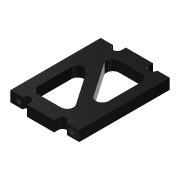
# Autodesk Inventor part: 前腕_サブフレーム_1_1
Saved by Autodesk Inventor 2017.3 (Build 213256000, 256)
## iProperties
Created: 2016-05-04
Part Number: 前腕_サブフレーム_1_1
Material: アセタール樹脂、黒
Document SubType Name: Modeling
Designer: hiroaki
Density: 1.425 g/cm^3
Appearance: 滑らか - 黒
Mass: 16.6655 g
Surface Area: 81.5563 cm^2
Volume: 11.6951 cm^3
Author: hiroaki
Autodesk Inventor part; units mm, degrees
ref_plane "YZ Plane" through (0, 0, 0) normal (1, 0, 0) x (0, 1, 0)
ref_plane "XZ Plane" through (0, 0, 0) normal (0, 1, 0) x (-1, 0, 0)
ref_plane "XY Plane" through (0, 0, 0) normal (0, 0, 1) x (1, 0, 0)
sketch "スケッチ1" plane through (0, 0, 0) normal (0, 0, 1) x (1, 0, 0)
  line L0 (-16.5, -21.65) -> (16.5, -21.65) construction
  line L1 (16.5, -21.65) -> (16.5, 21.65) construction
  line L2 (16.5, 21.65) -> (-16.5, 21.65) construction
  line L3 (-16.5, 21.65) -> (-16.5, -21.65) construction
  line L4 (-16.5, -21.65) -> (16.5, 21.65) construction
  line L5 (16.5, -21.65) -> (-16.5, 21.65) construction
  line L6 (-12.5, 21.65) -> (-12.5, -21.65) construction
  line L7 (0, 0) -> (0, 21.65) construction
  line L8 (0, 0) -> (-16.5, 0) construction
  line L9 (12.5, 21.65) -> (12.5, -21.65) construction
  line L10 (-16.5, -21.65) -> (-10.6, -21.65)
  line L11 (-6.5, 21.65) -> (-6.5, 23.65)
  line L12 (-6.5, 23.65) -> (6.5, 23.65)
  line L13 (6.5, 23.65) -> (6.5, 21.65)
  line L14 (10.6, 21.65) -> (16.5, 21.65)
  line L15 (16.5, 21.65) -> (16.5, -21.65)
  line L16 (16.5, -21.65) -> (10.6, -21.65)
  line L17 (-6.5, -21.65) -> (-6.5, -23.65)
  line L18 (-6.5, -23.65) -> (6.5, -23.65)
  line L19 (6.5, -23.65) -> (6.5, -21.65)
  arc A0 (-10.6, 21.65) -> (-6.5, 21.65) centre (-8.55, 21.65) ccw
  arc A1 (6.5, 21.65) -> (10.6, 21.65) centre (8.55, 21.65) ccw
  arc A2 (-6.5, -21.65) -> (-10.6, -21.65) centre (-8.55, -21.65) ccw
  arc A3 (10.6, -21.65) -> (6.5, -21.65) centre (8.55, -21.65) ccw
  line L20 (-16.5, -21.65) -> (-16.5, -16.65)
  line L21 (-16.5, -16.65) -> (-16.5, 21.65)
  line L22 (-10.6, 21.65) -> (-16.5, 21.65)
  line L23 (6.95, 24.476) -> (10.05, 24.476) construction
  line L24 (10.05, 24.476) -> (10.05, 13.3235) construction
  line L25 (10.05, 13.3235) -> (6.95, 13.3235) construction
  line L26 (6.95, 13.3235) -> (6.95, 24.476) construction
  line L27 (8.5, 24.476) -> (8.5, 13.3235) construction
  line L28 (-18.05, 24.476) -> (-14.95, 24.476) construction
  line L29 (-14.95, 24.476) -> (-14.95, 13.9945) construction
  line L30 (-14.95, 13.9945) -> (-18.05, 13.9945) construction
  line L31 (-18.05, 13.9945) -> (-18.05, 24.476) construction
  line L32 (-16.5, 24.476) -> (-16.5, 13.9945) construction
  dimension "d16" = 4
  dimension "d20" = 43.3
  dimension "d40" = 25
  dimension "d41" = 6
  dimension "d42" = 2.05
  dimension "d43" = 2
  dimension "d44" = 5
  dimension "d48" = 3.1
  dimension "d51" = 25
  dimension "d52" = 3.1
  dimension "d81" = 6
  constraints: 66 end point, 11 perpendicular, 8 midpoint, 8 point on circle, 6 parallel, 6 point on line, 5 collinear, 4 centre point, 4 horizontal, 4 horizontal alignment, 3 equal radius, 3 tangent, 2 symmetric about line, 2 vertical, 4 other
  measures "d16" distance between parallel lines of L3 L6
  measures "d20" distance of L2.end L0.start
  measures "d40" distance between parallel lines of L9 L6
  measures "d41" distance between parallel lines of L6 L17
  measures "d42" radius of A2
  measures "d43" distance between parallel lines of L0 L18
  measures "d44" distance from line of L10 L20.end
  measures "d48" distance of L23.start L23.end
  measures "d51" distance between parallel lines of L27 L32
  measures "d52" distance of L28.start L28.end
  measures "d81" distance between parallel lines of L11 L6
extrude "押し出し1" add sketch "スケッチ1" along normal blind 2.5
mirror "ミラー1" about plane through (0, 0, 0) normal (0, 0, -1) of "押し出し1"
sketch "スケッチ2" plane through (-16.5, -21.65, 2.5) normal (0, -1, 0) x (1, 0, 0)
  line L0 (0, -5) -> (0, 0)
  line L1 (10, -5) -> (23, -5) construction
  line L2 (16.5, -5) -> (16.5, 0) construction
  line L3 (10, 0) -> (23, 0) construction
  point P0 (16.5, -2.5)
  point P1 (4, -2.5)
  point P2 (29, -2.5)
  point P3 (0, -2.5)
  dimension "d26" = 4
  constraints: 4 end point, 3 midpoint, 2 horizontal alignment, 1 symmetric about line
  measures "d26" distance from line of point (4, -2.5) L0
hole "穴1" at (-12.5, -21.65, 0) at (12.5, -21.65, 0) direction (0, 1, 0) diameter 2.459 depth 2 thread size "M3x0.5" class "6H" standard "ISO Metric profile"
sketch "スケッチ4" plane through (10.6, 21.65, 2.5) normal (0, 1, 0) x (1, 0, 0)
  line L0 (5.9, 5) -> (5.9, 0) projected
  point P0 (-10.6, 2.5)
  point P1 (1.9, 2.5)
  point P2 (-23.1, 2.5)
  point P3 (5.9, 2.5)
  dimension "d53" = 4
  dimension "d54" = 25
  constraints: 2 horizontal alignment, 1 midpoint
  measures "d53" distance from line of point (1.9, 2.5) L0
  measures "d54" distance of point (-23.1, 2.5) point (1.9, 2.5)
hole "穴2" at (12.5, 21.65, 0) at (-12.5, 21.65, 0) direction (0, -1, 0) diameter 2.459 depth 2.5 thread size "M3x0.5" class "6H" standard "ISO Metric profile"
sketch "スケッチ6" plane through (0, 0, 2.5) normal (0, 0, 1) x (1, 0, 0)
  line L0 (10.6, -21.65) -> (16.5, -21.65) projected
  line L1 (16.5, -21.65) -> (16.5, 21.65) projected
  line L2 (16.5, 21.65) -> (10.6, 21.65) projected
  line L3 (-16.5, 21.65) -> (-16.5, -21.65) projected
  line L4 (11.5, 16.65) -> (11.5, -16.65) construction
  line L5 (11.5, -16.65) -> (-11.5, -16.65) construction
  line L6 (-11.5, -16.65) -> (-11.5, 12.251) construction
  line L7 (-11.5, 16.65) -> (11.5, 16.65) construction
  line L8 (11.5, -16.65) -> (-11.5, 16.65) construction
  line L9 (11.5, -12.251) -> (11.5, 16.65)
  line L10 (11.5, 16.65) -> (-8.4616, 16.65)
  line L11 (-8.4616, 16.65) -> (11.5, -12.251)
  line L12 (8.4616, -16.65) -> (-11.5, -16.65)
  line L13 (-11.5, -16.65) -> (-11.5, 12.251)
  line L14 (-11.5, 12.251) -> (8.4616, -16.65)
  point P0 (-20.5, -16.65)
  point P1 (0, 0)
  dimension "d72" = 5
  dimension "d73" = 5
  dimension "d74" = 5
  dimension "d75" = 5
  dimension "d76" = 5
  constraints: 22 end point, 4 collinear, 3 vertical, 2 horizontal, 2 parallel, 2 perpendicular, 1 point on line, 2 other
  measures "d72" distance between parallel lines of L7 L2
  measures "d73" distance between parallel lines of L0 L5
  measures "d74" distance between parallel lines of L1 L4
  measures "d76" distance between parallel lines of L14 L11
extrude "押し出し4" cut sketch "スケッチ6" against normal blind 10
fillet "フィレット3" radius 3 6 edges at (11.5, -12.251, 0) (8.4616, -16.65, 0) (-11.5, -16.65, 0) (11.5, 16.65, 0) (-8.4616, 16.65, 0) (-11.5, 12.251, 0)
equation "\"d40\" = d6"
equation "\"d53\" = d50"
equation "\"d54\" = d51"
equation "\"d73\" = d72"
equation "\"d74\" = d73"
equation "\"d75\" = d74"
equation "\"d76\" = d74"
equation "\"d4\" = 8"
equation "\"d6\" = 25"
equation "\"d50\" = 4"
